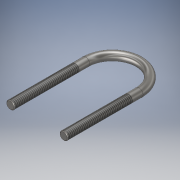
# Autodesk Inventor part: 0070.1 - Abraçadeira U Vergalhão bitola 1 polegada 80mm rosca 1 quarto
Saved by Autodesk Inventor 2019.4 (Build 234330000, 330)
## iProperties
Created: 2021-04-21
Part Number: 0070.1 - Abraçadeira U Vergalhão bitola 1 polegada 80mm rosca 1 quarto
Material: Aço, carbono
Document SubType Name: Modeling
Designer: Lattes
Density: 7.85 g/cm^3
Appearance: Semipolido
Author: Lattes
Autodesk Inventor part; units mm, degrees
ref_plane "YZ Plane" through (0, 0, 0) normal (1, 0, 0) x (0, 1, 0)
ref_plane "XZ Plane" through (0, 0, 0) normal (0, 1, 0) x (-1, 0, 0)
ref_plane "XY Plane" through (0, 0, 0) normal (0, 0, 1) x (1, 0, 0)
sketch "Esboço1" plane through (0, 0, 0) normal (0, 0, 1) x (1, 0, 0)
  circle A0 centre (0, 0) radius 3.175
  line L0 (20.5, 0) -> (20.5, 7.6069)
  dimension "d1" = 6.35
  constraints: 2 end point, 1 centre point, 1 coincident, 1 vertical
  measures "d1" diameter of A0
revolve "Revolução1" add sketch "Esboço1" angle 180 about axis through (20.5, 0, 0) along (0, -1, 0)
sketch "Esboço2" plane through (0, 0, 0) normal (0, 0, 1) x (1, 0, 0)
  circle A0 centre (0, 0) radius 3.175
  circle A1 centre (41, 0) radius 3.175 projected
  circle A2 centre (41, 0) radius 3.175
  constraints: 2 centre point, 2 coincident
extrude "Extrusão1" add sketch "Esboço2" along normal blind 58
thread "Rosca1" size "1/4-20 UNC" class "2A" standard "ANSI Unified Screw Threads" length 50 offset 8
thread "Rosca2" size "1/4-20 UNC" class "2A" standard "ANSI Unified Screw Threads" length 50
chamfer "Chanfro1" distance 0.5 angle 45 2 edges at (-3.175, 0, 58) (37.825, 0, 58)
